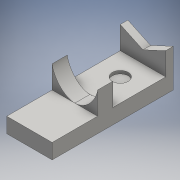
# Autodesk Inventor part: stand
Saved by Autodesk Inventor 2016 (Build 200138000, 138)
## iProperties
Created: 2015-12-26
Part Number: stand
Material: Generic
Document SubType Name: Modeling
Designer: gregg
Density: 1 g/cm^3
Appearance: Default
Author: gregg
Autodesk Inventor part; units mm, degrees
ref_plane "YZ Plane" through (0, 0, 0) normal (1, 0, 0) x (0, 1, 0)
ref_plane "XZ Plane" through (0, 0, 0) normal (0, 1, 0) x (-1, 0, 0)
ref_plane "XY Plane" through (0, 0, 0) normal (0, 0, 1) x (1, 0, 0)
sketch "Sketch1" plane through (0, 0, 0) normal (0, 0, 1) x (1, 0, 0)
  line L0 (0, 0) -> (30, 0)
  line L1 (30, 0) -> (30, -30)
  line L2 (30, -30) -> (0, -30)
  line L3 (0, -30) -> (0, 0)
  dimension "d2" = 30
  dimension "d3" = 30
  constraints: 8 end point, 2 parallel, 1 horizontal, 1 perpendicular
  measures "d2" distance of L1.end L2.end
  measures "d3" distance of L0.end L1.end
extrude "Extrusion1" add sketch "Sketch1" along normal blind 10
sketch "Sketch2" plane through (0, 0, 0) normal (0, 1, 0) x (1, 0, 0)
  line L0 (30, -10) -> (0, -10) projected
  line L1 (30, -10) -> (30, -25)
  line L2 (0, 0) -> (0, -10) projected
  line L3 (0, -25) -> (0, -10)
  spline S0 degree 4 poles (30, -25) (29.1667, -16.6667) (15, 3.8889) (0.8333, -16.6667) (0, -25) knots 0 0 0 0 0 1 1 1 1 1
  line L4 (15, -10) -> (30, -10) construction
  line L5 (15, -10) -> (0, -10) construction
  line L6 (0, -10) -> (5, -15) construction
  line L7 (5, -15) -> (25, -15) construction
  line L8 (30, -10) -> (25, -15) construction
  point P0 (24.1347, -10)
  point P1 (8.1347, -10)
  point P2 (15, -10)
  point P3 (0, -25)
  point P4 (30, -25)
  dimension "d16" = 15
  dimension "d18" = 0
  dimension "d19" = 5
  dimension "d20" = 5
  constraints: 14 end point, 3 equal length, 3 point on line, 1 collinear, 1 horizontal, 1 midpoint, 1 vertical, 8 other
  measures "d16" distance of L0.start L1.end
  measures "d18" distance from line of L0 L4.start
  measures "d19" distance from line of L0 L6.end
  measures "d20" distance from line of L3 L6.end
extrude "Extrusion2" add sketch "Sketch2" along normal blind 10
sketch "Sketch3" plane through (0, 0, 0) normal (0, 1, 0) x (1, 0, 0)
  line L0 (0, 0) -> (30, 0) projected
  line L1 (0, 0) -> (0, -10) projected
  line L2 (30, 0) -> (30, -10) projected
  line L3 (15, -10) -> (0, -10) projected
  line L4 (30, -10) -> (15, -10) projected
extrude "Extrusion3" add sketch "Sketch3" along normal blind 50
sketch "Sketch4" plane through (0, 50, 0) normal (0, 1, 0) x (1, 0, 0)
  line L0 (30, -10) -> (30, -25)
  line L1 (30, -25) -> (15, -18)
  line L2 (15, -18) -> (0, -25)
  line L3 (0, -25) -> (0, -10)
  line L4 (0, -10) -> (30, -10) projected
  line L5 (30, -10) -> (0, -10)
  dimension "d27" = 8
  dimension "d28" = 15
  constraints: 10 end point, 2 equal length, 1 horizontal, 1 parallel, 1 vertical
  measures "d27" distance from line of L4 L1.end
  measures "d28" distance of L3.end L2.end
extrude "Extrusion4" add sketch "Sketch4" against normal blind 5
sketch "Sketch5" plane through (0, 10, 10) normal (0, 0, 1) x (1, 0, 0)
  circle A0 centre (15, 20) radius 5.25
  line L0 (15, 20) -> (30, 20) construction
  line L1 (15, 20) -> (0, 20) construction
  line L2 (30, 0) -> (30, 35) construction
  line L3 (0, 0) -> (0, 35) construction
  line L4 (15, 0) -> (0, 0) construction
  point P0 (0, -10)
  point P1 (30, 40)
  point P2 (0, 40)
  dimension "d21" = 10.5
  dimension "d22" = 20
  constraints: 4 end point, 2 horizontal, 2 point on line, 1 centre point, 1 collinear
  measures "d21" diameter of A0
  measures "d22" distance between parallel lines of L1 L4
extrude "Extrusion5" cut sketch "Sketch5" against normal blind 2
body "Solid1"
